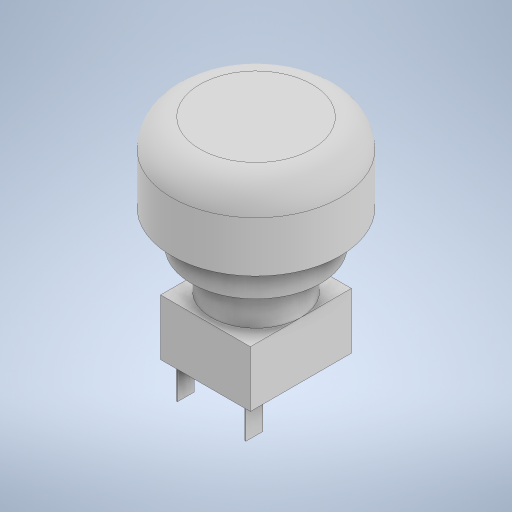
# Autodesk Inventor part: emergency_button
Saved by Autodesk Inventor 2024.1 (Build 281209000, 209)
## iProperties
Created: 2024-08-05
Part Number: emergency_button
Material: 一般
Document SubType Name: Modeling
Designer: hibik
Density: 1 g/cm^3
Appearance: 既定
Author: hibik
Autodesk Inventor part; units mm, degrees
ref_plane "YZ Plane" through (0, 0, 0) normal (1, 0, 0) x (0, 1, 0)
ref_plane "XZ Plane" through (0, 0, 0) normal (0, 1, 0) x (-1, 0, 0)
ref_plane "XY Plane" through (0, 0, 0) normal (0, 0, 1) x (1, 0, 0)
sketch "スケッチ1" plane through (0, 0, 0) normal (0, 1, 0) x (-1, 0, 0)
  circle A0 centre (0, 0) radius 8
  dimension "d0" = 16
  constraints: 1 centre point, 1 coincident
  measures "d0" diameter of A0
extrude "押し出し1" add sketch "スケッチ1" along normal blind 7
sketch "スケッチ2" plane through (0, 7, 0) normal (0, 1, 0) x (1, 0, 0)
  circle A0 centre (0, 0) radius 11.5
  dimension "d3" = 23
  constraints: 1 centre point, 1 coincident
  measures "d3" diameter of A0
extrude "押し出し2" add sketch "スケッチ2" along normal blind 6
sketch "スケッチ3" plane through (0, 13, 0) normal (0, 1, 0) x (1, 0, 0)
  circle A0 centre (0, 0) radius 15
  dimension "d6" = 30
  constraints: 1 centre point, 1 coincident
  measures "d6" diameter of A0
extrude "押し出し3" add sketch "スケッチ3" along normal blind 14
fillet "フィレット1" radius 5 1 edges at (-15, 27, 0)
sketch "スケッチ4" plane through (0, 0, 0) normal (0, -1, 0) x (1, 0, 0)
  line L0 (8, 9) -> (-8, 9)
  line L1 (-8, 9) -> (-8, -9)
  line L2 (-8, -9) -> (8, -9)
  line L3 (8, -9) -> (8, 9)
  circle A0 centre (0, 0) radius 10 projected
  line L4 (8, 9) -> (-8, -9) construction
  line L5 (-8, 9) -> (8, -9) construction
  dimension "d10" = 16
  dimension "d11" = 18
  constraints: 12 end point, 2 midpoint, 2 parallel, 1 horizontal, 1 perpendicular
  measures "d10" distance of L2.end L1.end
  measures "d11" distance of L1.end L0.end
extrude "押し出し4" add sketch "スケッチ4" along normal blind 10 contours L3 A0 L0 | A0 L3 L2 L1 L0 | A0 L1 L0 | L3 L2 A0 | A0 L2 L1
sketch "スケッチ5" plane through (0, -10, 0) normal (0, -1, 0) x (1, 0, 0)
  line L0 (-6, 8) -> (-6.2, 8)
  line L1 (-6.2, 8) -> (-6.2, 5)
  line L2 (-6.2, 5) -> (-6, 5)
  line L3 (-6, 5) -> (-6, 8)
  line L4 (6.2, 8) -> (6, 8)
  line L5 (6, 8) -> (6, 5)
  line L6 (6, 5) -> (6.2, 5)
  line L7 (6.2, 5) -> (6.2, 8)
  line L8 (0, -21) -> (0, 21) projected
  line L9 (8, 9) -> (-8, 9) projected
  point P0 (0, 0)
  point P1 (6.1, 8)
  dimension "d14" = 0.2
  dimension "d15" = 3
  dimension "d16" = 6
  dimension "d17" = 1
  constraints: 16 end point, 4 parallel, 2 equal length, 2 horizontal, 2 perpendicular, 1 collinear, 1 midpoint, 1 other
  measures "d14" distance of L0.start L0.end
  measures "d15" distance of L2.end L0.start
  measures "d16" distance between parallel lines of L5 L8
  measures "d17" distance from line of L9 point (6.1, 8)
extrude "押し出し5" add sketch "スケッチ5" along normal blind 6
